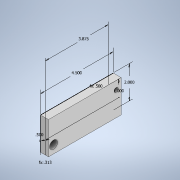
# Autodesk Inventor part: clolecton wheel holder
Saved by Autodesk Inventor 2021 (Build 250183000, 183)
## iProperties
Created: 2020-11-19
Part Number: clolecton wheel holder
Material: Generic
Document SubType Name: Modeling
Designer: gabe3
Density: 1 g/cm^3
Appearance: Default
Author: gabe3
Autodesk Inventor part; units mm, degrees
ref_plane "YZ Plane" through (0, 0, 0) normal (1, 0, 0) x (0, 1, 0)
ref_plane "XZ Plane" through (0, 0, 0) normal (0, 1, 0) x (-1, 0, 0)
ref_plane "XY Plane" through (0, 0, 0) normal (0, 0, 1) x (1, 0, 0)
sketch "Sketch2" plane through (0, 0, 0) normal (1, 0, 0) x (0, 1, 0)
  line L0 (0, 0) -> (50.8, 0)
  line L1 (50.8, 0) -> (50.8, -114.3)
  line L2 (50.8, -114.3) -> (0, -114.3)
  line L3 (0, -114.3) -> (0, 0)
  circle A0 centre (12.7, -7.9375) radius 6.35
  point P0 (38.1, -106.3625)
  dimension "d0" = 50.8
  dimension "d1" = 114.3
  dimension "d2" = 98.425
  dimension "d3" = 25.4
  dimension "d4" = 12.7
  dimension "d5" = 7.9375
  dimension "d15" = 12.7
  constraints: 8 end point, 2 parallel, 1 centre point, 1 coincident, 1 horizontal, 1 perpendicular
  measures "d0" distance of L1.end L2.end
  measures "d1" distance of L0.end L1.end
  measures "d2" vertical distance of point (12.7, -7.937) point (38.1, -106.363)
  measures "d3" horizontal distance of point (12.7, -7.937) point (38.1, -106.363)
  measures "d4" distance from line of L1 point (38.1, -106.363)
  measures "d5" distance from line of L0 point (12.7, -7.937)
  measures "d15" diameter of A0
extrude "Extrusion1" add sketch "Sketch2" along normal blind 12.7 contours L0 L1 L2 L3 | A0
hole "Hole1" at (0, 38.1, -106.3625) direction (1, 0, 0) diameter 6.35 depth 19.05 tip angle 118
hole "Hole2" at (0, 12.7, -7.9375) direction (1, 0, 0) diameter 12.7 depth 19.05 tip angle 118
equation "\"d4\" = -0.5 * d3 + 0.5 * d0"
equation "\"d5\" = -0.5 * d2 + 0.5 * d1"
body "Solid1"
